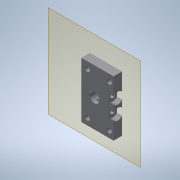
# Autodesk Inventor part: 30_Cube_Z_Focus_NEMA8_captive_micrometerscrewbase_v0
Saved by Autodesk Inventor 2022 (Build 260153000, 153)
## iProperties
Created: 2022-05-23
Part Number: 30_Cube_Z_Focus_NEMA8_captive_micrometerscrewbase_v0
Material: Generisch
Document SubType Name: Modeling
Designer: diederichbenedict
Density: 1 g/cm^3
Appearance: Vorgabe
Author: diederichbenedict
Autodesk Inventor part; units mm, degrees
ref_plane "YZ Plane" through (0, 0, 0) normal (1, 0, 0) x (0, 1, 0)
ref_plane "XZ Plane" through (0, 0, 0) normal (0, 1, 0) x (-1, 0, 0)
ref_plane "XY Plane" through (0, 0, 0) normal (0, 0, 1) x (1, 0, 0)
ref_plane "Arbeitsebene1" through (-0.0002, 0, 0) normal (0, 0, 1) x (1, 0, 0)
sketch "Skizze1" plane through (-0.0002, 0, 0) normal (0, 0, 1) x (1, 0, 0)
  circle A0 centre (13.85, 6.86) radius 1.5
  circle A1 centre (0.85, 31.86) radius 1.5
  circle A2 centre (13.85, 31.86) radius 1.5
  circle A3 centre (0.85, 6.86) radius 1.5
  circle A4 centre (5.0933, 19.36) radius 5.5
  line L0 (-3.07, 5.49) -> (-3.07, 33.23)
  line L1 (-3.07, 5.49) -> (-16.87, 5.49)
  line L2 (-16.87, 13.31) -> (-16.87, 5.49)
  line L3 (-16.8476, 13.31) -> (-16.87, 13.31)
  line L4 (-16.8476, 25.41) -> (-16.8476, 13.31)
  line L5 (-16.87, 25.41) -> (-16.8476, 25.41)
  line L6 (-16.87, 33.23) -> (-16.87, 25.41)
  line L7 (-3.07, 33.23) -> (-16.87, 33.23)
  line L8 (-16.87, 40.13) -> (-16.87, 44.21)
  line L9 (-20.77, 36.23) -> (-16.87, 40.13)
  line L10 (-24.85, 36.23) -> (-20.77, 36.23)
  line L11 (-24.85, 2.49) -> (-24.85, 36.23)
  line L12 (-20.77, 2.49) -> (-24.85, 2.49)
  line L13 (-16.87, -1.41) -> (-20.77, 2.49)
  line L14 (-16.87, -1.41) -> (-16.87, -5.49)
  line L15 (-16.87, -5.49) -> (16.87, -5.49)
  line L16 (16.87, -5.49) -> (16.87, -1.41)
  line L17 (20.77, 2.49) -> (16.87, -1.41)
  line L18 (24.85, 2.49) -> (20.77, 2.49)
  line L19 (24.85, 36.23) -> (24.85, 2.49)
  line L20 (20.77, 36.23) -> (24.85, 36.23)
  line L21 (16.87, 40.13) -> (20.77, 36.23)
  line L22 (16.87, 44.21) -> (16.87, 40.13)
  line L23 (-16.87, 44.21) -> (16.87, 44.21)
  line L24 (16.97, 36.33) -> (16.97, 2.39)
  line L25 (-16.97, 36.33) -> (16.97, 36.33) construction
  line L26 (-16.97, 2.39) -> (-16.97, 36.33)
  line L27 (16.97, 2.39) -> (-16.97, 2.39) construction
  line L28 (16.97, 2.39) -> (-16.97, 2.39)
  line L29 (16.47, 35.83) -> (16.47, 2.89)
  line L30 (16.47, 2.89) -> (-16.47, 2.89)
  line L31 (-16.47, 2.89) -> (-16.47, 35.83)
  line L32 (-16.47, 35.83) -> (16.47, 35.83)
  line L33 (-2.57, 35.83) -> (-2.57, 2.89)
  circle A5 centre (5.0933, 19.36) radius 3.505
  circle A6 centre (5.0933, 19.36) radius 3
  point P0 (0.0002, 0)
extrude "Extrusion1" add sketch "Skizze1" along normal blind 5 contours A4 | L33 L32 L29 L30 | A5
sketch "Skizze5" plane through (16.4698, 2.89, 0) normal (1, 0, 0) x (0, 0, -1)
  line L0 (-23, 19.975) -> (-13.08, 19.975)
  line L1 (-23, 12.965) -> (-13.08, 12.965)
  circle A0 centre (-2.5, 20.5313) radius 1.4
  circle A1 centre (-2.5, 12.3138) radius 1.4
  line L2 (0, 0) -> (0, 32.94) projected
  line L3 (0, 32.94) -> (-5, 32.94) projected
  line L4 (-5, 0) -> (-5, 32.94) projected
  line L5 (0, 0) -> (-5, 0) projected
  line L6 (-5, 13.47) -> (-5, 19.47) projected
  line L7 (0, 13.47) -> (0, 19.47) projected
  line L8 (-5, 32.94) -> (-5, 0) projected
  line L9 (-5, 0) -> (-5, 32.94) projected
  line L10 (-5, 2.47) -> (-5, 5.47) projected
  line L11 (-5, 27.47) -> (-5, 30.47) projected
  line L12 (-5, 27.47) -> (-5, 30.47) projected
  line L13 (-5, 2.47) -> (-5, 5.47) projected
  line L14 (-5, 13.47) -> (-5, 19.47) projected
  line L15 (-5, 19.47) -> (0, 19.47) projected
  line L16 (-5, 13.47) -> (0, 13.47) projected
  point P0 (0, -2.89)
  dimension "d19" = 2.8
  dimension "d20" = 2.8
  constraints: 4 end point, 2 centre point, 2 horizontal, 4 other
  measures "d19" diameter of A0
  measures "d20" diameter of A1
hole "Bohrung2" at (16.4698, 23.4213, 2.5) at (16.4698, 15.2038, 2.5) direction (-1, 0, 0) diameter 2.8 depth 30 counterbore diameter 6.5 counterbore depth 3
